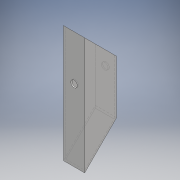
# Autodesk Inventor part: 車軸受け1
Saved by Autodesk Inventor 2018 (Build 220112000, 112)
## iProperties
Created: 2017-09-14
Part Number: 車軸受け1
Material: 一般
Document SubType Name: Modeling
Designer: mura5
Density: 1 g/cm^3
Appearance: 既定
Author: mura5
Autodesk Inventor part; units mm, degrees
ref_plane "YZ Plane" through (0, 0, 0) normal (1, 0, 0) x (0, 1, 0)
ref_plane "XZ Plane" through (0, 0, 0) normal (0, 1, 0) x (-1, 0, 0)
ref_plane "XY Plane" through (0, 0, 0) normal (0, 0, 1) x (1, 0, 0)
sketch "スケッチ1" plane through (0, 0, 0) normal (0, 0, 1) x (1, 0, 0)
  line L0 (-20, 30) -> (20, 30)
  line L1 (20, 30) -> (20, -30)
  line L2 (20, -30) -> (-20, -30)
  line L3 (-20, -30) -> (-20, 30)
  line L4 (-20, 30) -> (20, -30) construction
  line L5 (20, 30) -> (-20, -30) construction
  line L6 (17.7, 27.7) -> (-17.7, 27.7)
  line L7 (-17.7, 27.7) -> (-17.7, -27.7)
  line L8 (-17.7, -27.7) -> (17.7, -27.7)
  line L9 (17.7, -27.7) -> (17.7, 27.7)
  point P0 (0, 0)
  dimension "d0" = 40
  dimension "d1" = 60
  dimension "d2" = 2.3
  constraints: 20 end point, 4 parallel, 2 midpoint, 2 perpendicular, 1 horizontal, 3 other
  measures "d0" distance of L1.end L2.end
  measures "d1" distance of L0.end L1.end
  measures "d2" distance between parallel lines of L0 L6
extrude "押し出し1" add sketch "スケッチ1" along normal mid plane 220
chamfer "面取り1" distance 60 angle 45 2 edges at (0, 30, 110) (0, 30, -110)
sketch "スケッチ5" plane through (-20, -30, 110) normal (0, -1, 0) x (1, 0, 0)
  circle A0 centre (20, -85) radius 6.25
  point P0 (20, -110)
  dimension "d14" = 12.5
  dimension "d17" = 25
  constraints: 1 centre point, 1 coincident
  measures "d14" diameter of A0
  measures "d17" distance of point (20, -85) point (20, -110)
extrude "押し出し3" cut sketch "スケッチ5" against normal blind 250
